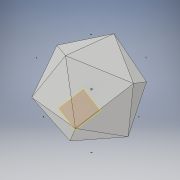
# Autodesk Inventor part: Icosahedron
Saved by Autodesk Inventor 2017 (Build 210142000, 142)
## iProperties
Created: 2017-08-14
Part Number: Icosahedron
Material: Generic
Document SubType Name: Modeling
Designer: Dale
Density: 1 g/cm^3
Appearance: Default
Author: Dale
## iProperties of the stored document Icosahedron_3DPrint.ipt
Created: 2017-08-14
Part Number: Icosahedron_3DPrint
Material: Generic
Document SubType Name: Modeling
Designer: Dale
Density: 1 g/cm^3
Appearance: Default
Author: Dale
Autodesk Inventor part; units mm, degrees
ref_plane "YZ Plane" through (0, 0, 0) normal (1, 0, 0) x (0, 1, 0)
ref_plane "XZ Plane" through (0, 0, 0) normal (0, 1, 0) x (-1, 0, 0)
ref_plane "XY Plane" through (0, 0, 0) normal (0, 0, 1) x (1, 0, 0)
sketch "Sketch1" plane through (0, 0, 0) normal (0, 0, 1) x (1, 0, 0)
  line L0 (0, 0) -> (40.45, 0)
  line L1 (40.45, 0) -> (40.45, 40.45)
  line L2 (40.45, 40.45) -> (0, 40.45)
  line L3 (0, 40.45) -> (0, 0)
  dimension "d1" = 40.45
  dimension "d2" = 40.45
  constraints: 8 end point, 2 parallel, 1 horizontal, 1 perpendicular
  measures "d1" distance of L2.end L0.start
  measures "d2" distance of L0.start L0.end
extrude "InitialCube" add sketch "Sketch1" along normal blind 40.45
sketch "Sketch2" plane through (40.45, 0, 0) normal (1, 0, 0) x (0, 0, -1)
  line L0 (-40.45, 0) -> (-40.45, 40.45)
  line L1 (-40.45, 40.45) -> (-25, 40.45)
  line L2 (-25, 40.45) -> (-40.45, 0)
  line L3 (0, 40.45) -> (-40.45, 40.45) projected
  line L4 (-40.45, 0) -> (-40.45, 40.45) projected
  point P0 (0, 0)
  dimension "d5" = 15.45
  constraints: 6 end point, 2 collinear, 1 perpendicular, 1 vertical
  measures "d5" distance of L0.end L1.end
extrude "YZ Trim" cut sketch "Sketch2" against normal blind 40.45
sketch "Sketch3" plane through (0, 0, 0) normal (0, -1, 0) x (1, 0, 0)
  line L0 (40.45, 0) -> (40.45, 40.45) projected
  line L1 (40.45, 40.45) -> (40.45, 0)
  line L2 (40.45, 0) -> (25, 40.45)
  line L3 (25, 40.45) -> (40.45, 40.45)
  point P0 (0, 0)
  dimension "d9" = 15.45
  constraints: 6 end point, 1 collinear, 1 perpendicular
  measures "d9" distance of L2.end L0.end
extrude "XZ Trim" cut sketch "Sketch3" against normal blind 40.45
sketch "Sketch4" plane through (0, 0, 0) normal (0, 0, -1) x (-1, 0, 0)
  line L0 (0, 40.45) -> (0, 0) projected
  line L1 (-40.45, 40.45) -> (0, 40.45) projected
  line L2 (0, 40.45) -> (-40.45, 40.45)
  line L3 (-40.45, 40.45) -> (-40.45, 25)
  line L4 (-40.45, 0) -> (-40.45, 40.45) projected
  line L5 (0, 40.45) -> (-40.45, 25)
  dimension "d12" = 15.45
  constraints: 6 end point, 1 horizontal, 1 point on line
  measures "d12" distance of L1.start L3.end
extrude "XY Trim" cut sketch "Sketch4" against normal blind 40.45
ref_plane "XYZ Work Plane" through (25, 0, 40.45) normal (0.5774, 0.5774, 0.5774) x (0.309, 0.5, -0.809)
sketch "Sketch6" plane through (25, 0, 40.45) normal (0.5774, 0.5774, 0.5774) x (0.309, 0.5, -0.809)
  line L0 (0, 0) -> (49.999, 0)
  line L1 (49.999, 0) -> (24.9995, 43.3004)
  line L2 (24.9995, 43.3004) -> (0, 0)
  point P0 (24.9995, 14.4335)
  constraints: 6 end point, 1 horizontal
extrude "XYZ Trim" cut sketch "Sketch6" along normal blind 12.5
mirror "Quarter Mirror" about plane through (20.225, 20.225, 0) normal (0, 0, -1) of "InitialCube", "XZ Trim", "XY Trim", "XYZ Trim", "YZ Trim"
mirror "Half Mirror" about plane through (0, 40.45, 0) normal (-1, 0, 0) of "InitialCube", "YZ Trim", "XZ Trim", "XY Trim", "XYZ Trim", "Quarter Mirror"
mirror "Full Mirror" about plane through (0, 0, 0) normal (0, -1, 0) of "Quarter Mirror", "InitialCube", "XZ Trim", "XY Trim", "XYZ Trim", "YZ Trim", "Half Mirror"
equation "\"d1\" = PhiLength"
equation "\"d2\" = PhiLength"
equation "\"d3\" = PhiLength"
equation "\"d5\" = SideDiff"
equation "\"d7\" = PhiLength"
equation "\"d9\" = SideDiff"
equation "\"d10\" = PhiLength"
equation "\"d12\" = SideDiff"
equation "\"d13\" = PhiLength"
equation "\"d16\" = 0.5 * SideLength"
equation "\"SideLength\" = 25"
equation "\"PhiLength\" = 1.618 * SideLength"
equation "\"SideDiff\" = PhiLength - SideLength"
body "Solid1"
